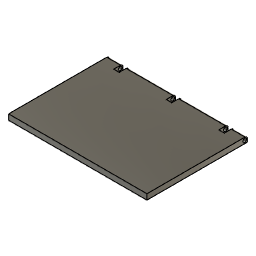
桶盖 (Autodesk Fusion 360 design; units mm, degrees)
part number: 2025-05-27-14-07-02-721
Autodesk Fusion 360 part; units mm, degrees
sketch "草图1" plane through (0, 0, 13.3714) normal (0, 0, 1) x (-1, 0, 0)
  line L0 (10.9987, -232.8503) -> (25.9987, -232.8503)
  line L1 (25.9987, -232.8503) -> (25.9987, -126.3503)
  line L2 (25.9987, -126.3503) -> (-124.0013, -126.3503)
  line L3 (-124.0013, -126.3503) -> (-124.0013, -232.8503)
  line L4 (-124.0013, -232.8503) -> (-109.0013, -232.8503)
  line L5 (-109.0013, -232.8503) -> (-109.0013, -225.3503)
  line L6 (-109.0013, -225.3503) -> (-103.0013, -225.3503)
  line L7 (-103.0013, -225.3503) -> (-103.0013, -232.8503)
  line L8 (-103.0013, -232.8503) -> (-52.0013, -232.8503)
  line L9 (-52.0013, -232.8503) -> (-52.0013, -225.3503)
  line L10 (-52.0013, -225.3503) -> (-46.0013, -225.3503)
  line L11 (-46.0013, -225.3503) -> (-46.0013, -232.8503)
  line L12 (-46.0013, -232.8503) -> (4.9987, -232.8503)
  line L13 (4.9987, -232.8503) -> (4.9987, -225.3503)
  line L14 (4.9987, -225.3503) -> (10.9987, -225.3503)
  line L15 (10.9987, -225.3503) -> (10.9987, -232.8503)
  line L16 (-114.0013, -225.3503) -> (-127.4522, -225.3503)
  line L17 (-127.4522, -225.3503) -> (-127.4522, -236.557)
  line L18 (-127.4522, -236.557) -> (-114.0013, -236.557)
  line L19 (-114.0013, -236.557) -> (-114.0013, -225.3503)
  line L20 (-98.0013, -225.3503) -> (-57.0013, -225.3503)
  line L21 (-57.0013, -225.3503) -> (-57.0013, -239)
  line L22 (-57.0013, -239) -> (-98.0013, -239)
  line L23 (-98.0013, -239) -> (-98.0013, -225.3503)
  line L24 (-41.0013, -225.3503) -> (-0.0013, -225.3503)
  line L25 (-0.0013, -225.3503) -> (-0.0013, -240)
  line L26 (-0.0013, -240) -> (-41.0013, -240)
  line L27 (-41.0013, -240) -> (-41.0013, -225.3503)
  line L28 (15.9987, -225.3503) -> (29.1278, -225.3503)
  line L29 (29.1278, -225.3503) -> (29.1278, -239)
  line L30 (29.1278, -239) -> (15.9987, -239)
  line L31 (15.9987, -239) -> (15.9987, -225.3503)
  dimension "d1" = 5
  dimension "d2" = 5
  dimension "d3" = 5
  dimension "d4" = 5
  dimension "d5" = 5
  dimension "d6" = 5
  constraint horizontal L16
  constraint vertical L17
  constraint horizontal L18
  constraint vertical L19
  constraint collinear L6 L16
  constraint horizontal L20
  constraint vertical L21
  constraint horizontal L22
  constraint vertical L23
  constraint horizontal L24
  constraint vertical L25
  constraint horizontal L26
  constraint vertical L27
  constraint horizontal L28
  constraint vertical L29
  constraint horizontal L30
  constraint vertical L31
  measures "d1" distance of L5 L19
  measures "d2" distance of L7 L23
  measures "d3" distance of L9 L21
  measures "d4" distance of L11 L27
  measures "d5" distance of L13 L25
  measures "d6" distance of L15 L31
sketch "草图2" plane through (150, 0, 0) normal (1, 0, 0) x (0, 1, 0)
  line L0 (0, 100) -> (109, 100)
  line L1 (109, 100) -> (109, 106)
  line L2 (109, 106) -> (0, 106)
  line L3 (0, 106) -> (0, 100)
  circle A0 centre (106, 103) radius 2
  dimension "d7" = 4
  dimension "d8" = 3
  dimension "d9" = 3
  measures "d7" diameter of A0
  measures "d8" distance of L1 A0.centre
  measures "d9" distance of L2 A0.centre
sketch "草图3" plane through (0, 0, 100) normal (0, 0, 1) x (-1, 0, 0)
  line L0 (-3, -29) -> (0, -29)
  line L1 (0, -29) -> (0, 0)
  line L2 (0, 0) -> (-63, 0)
  line L3 (-63, 0) -> (-63, -3)
  line L4 (-63, -3) -> (-3, -3)
  line L5 (-3, -3) -> (-3, -29)
  line L6 (0, -109) -> (-150, -109)
  line L7 (-150, -109) -> (-150, 0)
  line L8 (-150, 0) -> (0, 0)
  line L9 (0, 0) -> (0, -109)
  dimension "d10" = 150
  dimension "d11" = 109
  constraint horizontal L6
  constraint vertical L7
  constraint horizontal L8
  constraint vertical L9
  constraint coincident L1.end L2.start
  measures "d10" distance of L6.start L6.end
  measures "d11" distance of L6.start L1.end
sketch "草图4" plane through (0, 0, 106) normal (0, 0, 1) x (-1, 0, 0)
  line L0 (0, 0) -> (-150, 0)
  line L1 (-150, 0) -> (-150, -109)
  line L2 (-150, -109) -> (0, -109)
  line L3 (0, -109) -> (0, 0)
  line L4 (-135, -99) -> (-129, -99)
  line L5 (-129, -99) -> (-129, -109)
  line L6 (-129, -109) -> (-135, -109)
  line L7 (-135, -109) -> (-135, -99)
  line L8 (-78, -99) -> (-72, -99)
  line L9 (-72, -99) -> (-72, -109)
  line L10 (-72, -109) -> (-78, -109)
  line L11 (-78, -109) -> (-78, -99)
  line L12 (-21, -99) -> (-15, -99)
  line L13 (-15, -99) -> (-15, -109)
  line L14 (-15, -109) -> (-21, -109)
  line L15 (-21, -109) -> (-21, -99)
  dimension "d12" = 6
  dimension "d13" = 10
  dimension "d14" = 15
  dimension "d15" = 6
  dimension "d16" = 10
  dimension "d17" = 6
  dimension "d18" = 10
  dimension "d19" = 72
  dimension "d20" = 15
  constraint horizontal L4
  constraint vertical L5
  constraint horizontal L6
  constraint vertical L7
  constraint collinear L2 L6
  constraint horizontal L8
  constraint vertical L9
  constraint horizontal L10
  constraint vertical L11
  constraint horizontal L12
  constraint vertical L13
  constraint horizontal L14
  constraint vertical L15
  constraint collinear L2 L10
  constraint collinear L2 L14
  measures "d12" distance of L4.start L4.end
  measures "d13" distance of L4.start L6.end
  measures "d14" distance of L1 L7
  measures "d15" distance of L8.start L8.end
  measures "d16" distance of L8.start L10.end
  measures "d17" distance of L12.start L12.end
  measures "d18" distance of L12.start L14.end
  measures "d19" distance of L1 L11
  measures "d20" distance of L3 L13
extrude "拉伸1" add sketch "草图3" along normal blind 6
extrude "拉伸2" cut sketch "草图4" against normal blind 10 contours L2 L12 L13 L14 L15 | L2 L4 L5 L6 L7 | L2 L8 L9 L10 L11
extrude "拉伸3" cut sketch "草图2" against normal blind 170 contours A0
fillet "圆角1" radius 2.5 4 edges at (142.5, 109, 106) (103.5, 109, 106) (46.5, 109, 106) (7.5, 109, 106)
extrude "拉伸4" cut sketch "草图1" against normal blind 25 contours L0 L1 L28 L31 | L0 L1 L28 L29 L30 L31 | L12 L25 L26 L27 | L12 L24 L25 L27 | L3 L4 L16 L19 | L3 L4 L16 L17 L18 L19 | L8 L21 L22 L23 | L8 L20 L21 L23
